Autodesk Inventor part; units mm, degrees
(part 2 of 2)
sketch "Sketch26" plane through (0, 0, 0) normal (0, -1, 0) x (1, 0, 0)
  line L0 (81.6764, -211.0248) -> (81.6764, -203.0248)
  line L1 (72.0084, -212.0248) -> (80.6764, -212.0248)
  arc A0 (80.6764, -212.0248) -> (81.6764, -211.0248) centre (80.6764, -211.0248) ccw
  line L2 (80.6764, -211.0248) -> (80.6764, -219.0248)
  line L3 (80.6764, -219.0248) -> (180.6764, -219.0248)
  line L4 (80.6764, -219.0248) -> (85.6764, -219.0248)
  line L5 (85.6764, -219.0248) -> (85.6764, -69.0248)
  line L6 (85.6764, -69.0248) -> (180.6764, -219.0248)
  ellipse E0 centre (0, -304.8) end of major axis (0, -542.544) minor radius 177.8 (-124.461, -474.5818) -> (124.461, -474.5818) ccw projected
  line L7 (0, -542.544) -> (0, -67.056)
  ellipse E1 centre (0, -304.8) end of major axis (0, -542.544) minor radius 177.8 (124.461, -135.0182) -> (-124.461, -135.0182) ccw projected
  line L8 (0, -304.8) -> (-48.9321, -304.8)
  line L9 (81.6764, -398.5752) -> (81.6764, -406.5752)
  line L10 (72.0084, -397.5752) -> (80.6764, -397.5752)
  arc A1 (81.6764, -398.5752) -> (80.6764, -397.5752) centre (80.6764, -398.5752) ccw
  line L11 (80.6764, -398.5752) -> (80.6764, -390.5752)
  line L12 (80.6764, -390.5752) -> (180.6764, -390.5752)
  line L13 (80.6764, -390.5752) -> (85.6764, -390.5752)
  line L14 (85.6764, -390.5752) -> (85.6764, -540.5752)
  line L15 (85.6764, -540.5752) -> (180.6764, -390.5752)
  line L16 (-81.6764, -211.0248) -> (-81.6764, -203.0248)
  line L17 (-72.0084, -212.0248) -> (-80.6764, -212.0248)
  arc A2 (-81.6764, -211.0248) -> (-80.6764, -212.0248) centre (-80.6764, -211.0248) ccw
  line L18 (-80.6764, -211.0248) -> (-80.6764, -219.0248)
  line L19 (-80.6764, -219.0248) -> (-180.6764, -219.0248)
  line L20 (-80.6764, -219.0248) -> (-85.6764, -219.0248)
  line L21 (-85.6764, -219.0248) -> (-85.6764, -69.0248)
  line L22 (-85.6764, -69.0248) -> (-180.6764, -219.0248)
  line L23 (-81.6764, -398.5752) -> (-81.6764, -406.5752)
  line L24 (-72.0084, -397.5752) -> (-80.6764, -397.5752)
  arc A3 (-80.6764, -397.5752) -> (-81.6764, -398.5752) centre (-80.6764, -398.5752) ccw
  line L25 (-80.6764, -398.5752) -> (-80.6764, -390.5752)
  line L26 (-80.6764, -390.5752) -> (-85.6764, -390.5752)
  line L27 (-85.6764, -390.5752) -> (-85.6764, -540.5752)
  line L28 (-85.6764, -540.5752) -> (-180.6764, -390.5752)
  line L29 (-80.6764, -390.5752) -> (-180.6764, -390.5752)
  point P0 (0, 0)
  dimension "d215" = 8
  dimension "d216" = 100
  dimension "d217" = 5
  dimension "d218" = 150
  constraints: 60 end point, 27 symmetric about line, 8 point on circle, 4 centre point, 4 point on line, 3 vertical, 2 horizontal, 2 perpendicular, 13 other
  measures "d215" distance of L2.start L2.end
  measures "d216" distance of L2.end L3.end
  measures "d217" distance of L2.end L4.end
  measures "d218" distance of L4.end L5.end
extrude "Extrusion32" cut sketch "Sketch26" against normal blind 10
fillet "Fillet2" radius 20 8 edges at (85.6764, 3.175, -96.4785) (152.3368, 3.175, -219.0248) (152.3368, 3.175, -390.5752) (85.6764, 3.175, -513.1215) (-85.6764, 3.175, -513.1215) (-152.3368, 3.175, -390.5752) (-152.3368, 3.175, -219.0248) (-85.6764, 3.175, -96.4785)
fillet "Fillet3" radius 5 4 edges at (-85.6764, 3.175, -219.0248) (-85.6764, 3.175, -390.5752) (85.6764, 3.175, -390.5752) (85.6764, 3.175, -219.0248)
sketch "Sketch29" plane through (0, 6.35, 0) normal (0, 1, 0) x (1, 0, 0)
  line L0 (0, 357.742) -> (0, 329.1998)
  circle A0 centre (-32.385, 290.167) radius 1.5
  circle A1 centre (-32.385, 297.817) radius 1.5
  circle A2 centre (32.385, 290.167) radius 1.5
  circle A3 centre (32.385, 297.817) radius 1.5
  line L1 (-33.885, 290.167) -> (-33.885, 292.167)
  line L2 (-33.885, 292.167) -> (-33.885, 288.167)
  line L3 (-33.885, 297.817) -> (-33.885, 299.817)
  line L4 (-33.885, 297.817) -> (-33.885, 295.817)
  line L5 (-33.885, 288.167) -> (-30.885, 288.167)
  line L6 (-30.885, 288.167) -> (-30.885, 292.167)
  line L7 (-30.885, 292.167) -> (-33.885, 292.167)
  line L8 (-33.885, 292.167) -> (-33.885, 288.167)
  line L9 (-33.885, 295.817) -> (-30.885, 295.817)
  line L10 (-30.885, 295.817) -> (-30.885, 299.817)
  line L11 (-30.885, 299.817) -> (-33.885, 299.817)
  line L12 (-33.885, 299.817) -> (-33.885, 295.817)
  circle A4 centre (-32.385, 288.167) radius 1.5
  circle A5 centre (-32.385, 292.167) radius 1.5
  circle A6 centre (-32.385, 295.817) radius 1.5
  circle A7 centre (-32.385, 299.817) radius 1.5
  circle A8 centre (32.385, 290.167) radius 1.5
  circle A9 centre (32.385, 297.817) radius 1.5
  line L13 (33.885, 290.167) -> (33.885, 292.167)
  line L14 (33.885, 292.167) -> (33.885, 288.167)
  line L15 (33.885, 297.817) -> (33.885, 299.817)
  line L16 (33.885, 297.817) -> (33.885, 295.817)
  line L17 (33.885, 288.167) -> (30.885, 288.167)
  line L18 (30.885, 288.167) -> (30.885, 292.167)
  line L19 (30.885, 292.167) -> (33.885, 292.167)
  line L20 (33.885, 292.167) -> (33.885, 288.167)
  line L21 (33.885, 295.817) -> (30.885, 295.817)
  line L22 (30.885, 295.817) -> (30.885, 299.817)
  line L23 (30.885, 299.817) -> (33.885, 299.817)
  line L24 (33.885, 299.817) -> (33.885, 295.817)
  circle A10 centre (32.385, 288.167) radius 1.5
  circle A11 centre (32.385, 292.167) radius 1.5
  circle A12 centre (32.385, 295.817) radius 1.5
  circle A13 centre (32.385, 299.817) radius 1.5
  point P0 (0, 0)
  dimension "d235" = 2
  dimension "d236" = 4
  dimension "d237" = 2
  dimension "d238" = 2
  constraints: 50 end point, 19 symmetric about line, 8 horizontal alignment, 8 vertical, 6 centre point, 4 midpoint, 4 parallel, 4 point on circle, 4 point on line, 2 horizontal, 2 perpendicular, 1 tangent, 25 other
  measures "d235" distance of L1.start L1.end
  measures "d236" distance of L1.end L2.end
  measures "d237" distance of L3.start L3.end
  measures "d238" distance of L4.start L4.end
extrude "Extrusion33" cut sketch "Sketch29" against normal blind 10
sketch "Sketch30" plane through (0, 6.35, 0) normal (0, 1, 0) x (1, 0, 0)
  circle A0 centre (-56.7479, 237.5409) radius 1.25
  circle A1 centre (0, 237.056) radius 41.5 projected
  line L0 (0, 278.556) -> (0, 293.806)
  line L1 (-14.9781, 275.7588) -> (-20.8852, 289.8183)
  circle A2 centre (0, 237.056) radius 41.5
  line L2 (14.9781, 275.7588) -> (20.8852, 289.8183)
  circle A3 centre (-20.8852, 289.8183) radius 1.5
  circle A4 centre (20.8852, 289.8183) radius 1.5
  line L3 (0, 237.056) -> (67.6789, 237.056)
  circle A5 centre (0, 237.056) radius 41.5
  line L4 (0, 195.556) -> (0, 180.306)
  line L5 (-14.9781, 198.3532) -> (-20.8852, 184.2937)
  circle A6 centre (0, 237.056) radius 41.5
  line L6 (14.9781, 198.3532) -> (20.8852, 184.2937)
  circle A7 centre (-20.8852, 184.2937) radius 1.5
  circle A8 centre (20.8852, 184.2937) radius 1.5
  line L7 (31.588, 263.9716) -> (42.1224, 274.9983)
  circle A9 centre (42.1224, 274.9983) radius 1.5
  circle A10 centre (0, 237.056) radius 41.5
  circle A11 centre (0, 237.056) radius 41.5
  circle A12 centre (0, 237.056) radius 41.5
  circle A13 centre (0, 237.056) radius 41.5
  line L8 (-31.588, 263.9716) -> (-42.1224, 274.9983)
  circle A14 centre (-42.1224, 274.9983) radius 1.5
  point P0 (0, 0)
  dimension "d241" = 15.25
  dimension "d242" = 15.25
  dimension "d243" = 3
  dimension "d244" = 3
  dimension "d245" = 15.25
  dimension "d246" = 3
  constraints: 18 end point, 13 symmetric about line, 12 centre point, 6 coincident, 6 point on circle, 4 line through centre, 1 horizontal, 1 vertical, 14 other
  measures "d241" distance of L0.start L0.end
  measures "d242" distance of L1.start L1.end
  measures "d243" diameter of A3
  measures "d244" diameter of A4
  measures "d245" distance of L7.start L7.end
  measures "d246" diameter of A9
extrude "Extrusion34" cut sketch "Sketch30" against normal blind 10 contours A8 | A7 | A14 | A9
sketch "Sketch31" plane through (0, 0, 0) normal (0, -1, 0) x (1, 0, 0)
  line L0 (13.2, -423.6628) -> (13.2, -352.742) projected
  line L1 (13.2, -352.742) -> (16.2, -352.742)
  line L2 (16.2, -352.742) -> (16.2, -423.6628)
  line L3 (16.2, -423.6628) -> (13.2, -423.6628)
  line L4 (13.2, -423.6628) -> (13.2, -352.742)
  line L5 (13.2, -352.742) -> (-13.2, -352.742) projected
  line L6 (0, -352.742) -> (0, -346.4398)
  line L7 (-13.2, -423.6628) -> (-13.2, -352.742)
  line L8 (-13.2, -352.742) -> (-16.2, -352.742)
  line L9 (-16.2, -352.742) -> (-16.2, -423.6628)
  line L10 (-16.2, -423.6628) -> (-13.2, -423.6628)
  line L11 (-13.2, -423.6628) -> (-13.2, -352.742)
  line L12 (-13.2, -352.742) -> (13.2, -352.742)
  point P0 (0, 0)
  dimension "d254" = 3
  constraints: 22 end point, 6 symmetric about line, 2 parallel, 1 horizontal, 1 midpoint, 1 perpendicular, 1 vertical
  measures "d254" distance of L2.end L3.end
extrude "Extrusion35" cut sketch "Sketch31" against normal blind 10
sketch "Sketch32" plane through (0, 6.35, 0) normal (0, 1, 0) x (1, 0, 0)
  circle A0 centre (-25.9, 409.3128) radius 1.25
  circle A1 centre (-19.2, 409.3128) radius 1.25
  circle A2 centre (-25.9, 367.092) radius 1.25
  circle A3 centre (-19.2, 367.092) radius 1.25
  circle A4 centre (-19.2, 409.3128) radius 1.5
  circle A5 centre (-25.9, 409.3128) radius 1.5
  circle A6 centre (-25.9, 367.092) radius 1.5
  circle A7 centre (-19.2, 367.092) radius 1.5
  circle A8 centre (29.368, 370.8612) radius 1.25
  circle A9 centre (29.368, 415.7152) radius 1.25
  circle A10 centre (29.368, 415.7152) radius 1.5
  circle A11 centre (29.368, 370.8612) radius 1.5
  point P0 (0, 0)
  dimension "d257" = 3
  dimension "d258" = 3
  dimension "d259" = 3
  dimension "d260" = 3
  dimension "d263" = 3
  dimension "d264" = 3
  constraints: 12 centre point, 6 coincident, 12 other
  measures "d257" diameter of A4
  measures "d258" diameter of A5
  measures "d259" diameter of A6
  measures "d260" diameter of A7
  measures "d263" diameter of A10
  measures "d264" diameter of A11
extrude "Extrusion36" cut sketch "Sketch32" against normal blind 10 contours A0 | A1 | A2 | A3 | A4 | A5 | A6 | A7 | A8 | A9 | A10 | A11
sketch "Sketch33" plane through (0, 0, 0) normal (0, -1, 0) x (1, 0, 0)
  circle A0 centre (9.275, -529.719) radius 1.25
  circle A1 centre (-9.275, -529.719) radius 1.25
  circle A2 centre (-11.1, -519.544) radius 1.25
  circle A3 centre (-11.1, -511.544) radius 1.25
  circle A4 centre (11.1, -519.544) radius 1.25
  circle A5 centre (11.1, -511.544) radius 1.25
  circle A6 centre (-9.275, -529.719) radius 1.5
  circle A7 centre (9.275, -529.719) radius 1.5
  circle A8 centre (11.1, -519.544) radius 1.5
  circle A9 centre (11.1, -511.544) radius 1.5
  circle A10 centre (-11.1, -519.544) radius 1.5
  circle A11 centre (-11.1, -511.544) radius 1.5
  point P0 (0, 0)
  dimension "d265" = 3
  dimension "d266" = 3
  dimension "d267" = 3
  dimension "d268" = 3
  dimension "d269" = 3
  dimension "d270" = 3
  constraints: 12 centre point, 6 coincident, 8 other
  measures "d265" diameter of A6
  measures "d266" diameter of A7
  measures "d267" diameter of A8
  measures "d268" diameter of A9
  measures "d269" diameter of A10
  measures "d270" diameter of A11
extrude "Extrusion37" cut sketch "Sketch33" against normal blind 10 contours A0 | A1 | A2 | A3 | A4 | A5 | A6 | A7 | A8 | A9 | A10 | A11
sketch "Sketch34" plane through (0, 6.35, 0) normal (0, 1, 0) x (1, 0, 0)
  circle A0 centre (-37.6554, 463.12) radius 1.5
  circle A1 centre (-31.4515, 472.62) radius 1.5
  circle A2 centre (-37.6554, 483.332) radius 1.5
  circle A3 centre (-31.4515, 494.044) radius 1.5
  circle A4 centre (-37.6554, 503.544) radius 1.5
  circle A5 centre (-10.3593, 472.62) radius 1.5
  circle A6 centre (-4.1554, 463.12) radius 1.5
  circle A7 centre (-4.1554, 483.332) radius 1.5
  circle A8 centre (-10.3593, 494.044) radius 1.5
  circle A9 centre (-4.1554, 503.544) radius 1.5
  line L0 (0, 423.6628) -> (0, 542.544)
  circle A10 centre (-37.6554, 463.12) radius 1.75
  circle A11 centre (-31.4515, 472.62) radius 1.75
  circle A12 centre (-37.6554, 483.332) radius 1.75
  circle A13 centre (-31.4515, 494.044) radius 1.75
  circle A14 centre (-37.6554, 503.544) radius 1.75
  circle A15 centre (-10.3593, 472.62) radius 1.75
  circle A16 centre (-4.1554, 463.12) radius 1.75
  circle A17 centre (-4.1554, 483.332) radius 1.75
  circle A18 centre (-10.3593, 494.044) radius 1.75
  circle A19 centre (-4.1554, 503.544) radius 1.75
  circle A20 centre (37.6554, 463.12) radius 1.5
  circle A21 centre (31.4515, 472.62) radius 1.5
  circle A22 centre (37.6554, 483.332) radius 1.5
  circle A23 centre (11.1, 519.544) radius 1.5
  circle A24 centre (11.1, 511.544) radius 1.5
  circle A25 centre (45.5449, 473.4142) radius 1.75
  circle A26 centre (31.4515, 494.044) radius 1.5
  circle A27 centre (37.6554, 503.544) radius 1.5
  circle A28 centre (10.3593, 472.62) radius 1.5
  circle A29 centre (4.1554, 463.12) radius 1.5
  circle A30 centre (4.1554, 483.332) radius 1.5
  circle A31 centre (10.3593, 494.044) radius 1.5
  circle A32 centre (4.1554, 503.544) radius 1.5
  circle A33 centre (37.6554, 463.12) radius 1.75
  circle A34 centre (31.4515, 472.62) radius 1.75
  circle A35 centre (37.6554, 483.332) radius 1.75
  circle A36 centre (31.4515, 494.044) radius 1.75
  circle A37 centre (37.6554, 503.544) radius 1.75
  circle A38 centre (10.3593, 472.62) radius 1.75
  circle A39 centre (4.1554, 463.12) radius 1.75
  circle A40 centre (4.1554, 483.332) radius 1.75
  circle A41 centre (10.3593, 494.044) radius 1.75
  circle A42 centre (4.1554, 503.544) radius 1.75
  point P0 (0, 0)
  point P1 (-11.1, 519.544)
  point P2 (-11.1, 511.544)
  point P3 (-45.5449, 473.4142)
  dimension "d273" = 3.5
  dimension "d274" = 3.5
  dimension "d275" = 3.5
  dimension "d276" = 3.5
  dimension "d277" = 3.5
  dimension "d278" = 3.5
  dimension "d279" = 3.5
  dimension "d280" = 3.5
  dimension "d281" = 3.5
  dimension "d282" = 3.5
  constraints: 43 centre point, 23 symmetric about line, 20 coincident, 2 end point, 40 other
  measures "d273" diameter of A10
  measures "d274" diameter of A11
  measures "d275" diameter of A12
  measures "d276" diameter of A13
  measures "d277" diameter of A14
  measures "d278" diameter of A15
  measures "d279" diameter of A16
  measures "d280" diameter of A17
  measures "d281" diameter of A18
  measures "d282" diameter of A19
extrude "Extrusion38" cut sketch "Sketch34" against normal blind 10 contours A0 | A1 | A2 | A3 | A4 | A5 | A6 | A7 | A8 | A9 | A10 | A11 | A12 | A13 | A14 | A15 | A16 | A17 | A18 | A19 | A20 | A21 | A22 | A26 | A27 | A28 | A29 | A30 | A31 | A32 | A33 | A34 | A35 | A36 | A37 | A38 | A39 | A40 | A41 | A42
sketch "Sketch35" plane through (0, 6.35, 0) normal (0, 1, 0) x (1, 0, 0)
  circle A0 centre (-0.1147, 432.1266) radius 1.375
  circle A1 centre (-0.1147, 432.1266) radius 1.75
  point P0 (0, 0)
  dimension "d285" = 3.5
  constraints: 2 centre point, 1 coincident, 2 other
  measures "d285" diameter of A1
extrude "Extrusion39" cut sketch "Sketch35" against normal blind 10 contours A0 | A1
fillet "Fillet4" radius 2 4 edges at (-16.2, 3.175, -352.742) (16.2, 3.175, -352.742) (-16.2, 3.175, -423.6628) (16.2, 3.175, -423.6628)
body "Solid2"
